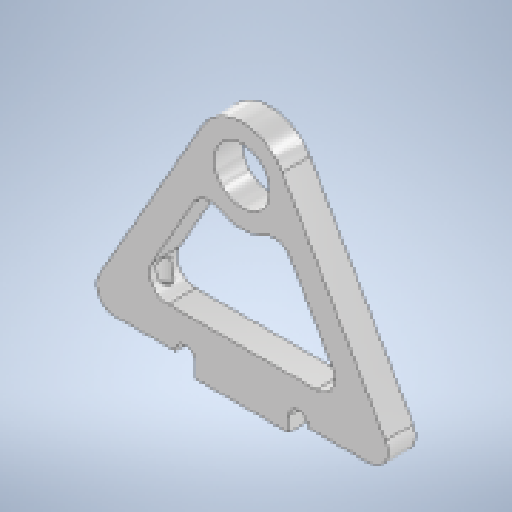
# Autodesk Inventor part: kosipiti
Saved by Autodesk Inventor 2025.1 (Build 291241000, 241)
## iProperties
Created: 2024-09-01
Part Number: kosipiti
Material: アルミニウム 2014-T4
Document SubType Name: Modeling
Designer: right
Density: 2.8 g/cm^3
Appearance: サテン
Mass: 2.87521 g
Surface Area: 14.5004 cm^2
Volume: 1.02686 cm^3
Author: right
Autodesk Inventor part; units mm, degrees
ref_plane "YZ Plane" through (0, 0, 0) normal (1, 0, 0) x (0, 1, 0)
ref_plane "XZ Plane" through (0, 0, 0) normal (0, 1, 0) x (-1, 0, 0)
ref_plane "XY Plane" through (0, 0, 0) normal (0, 0, 1) x (1, 0, 0)
sketch "スケッチ1" plane through (0, 0, 0) normal (0, 0, 1) x (1, 0, 0)
  circle A0 centre (0, 0) radius 3
  circle A1 centre (0, 0) radius 5
  line L0 (-5, -20) -> (5, -20)
  line L1 (5, -20) -> (5, -21.5)
  line L2 (5, -21.5) -> (-5, -21.5)
  line L3 (-5, -21.5) -> (-5, -20)
  circle A2 centre (-6.1, -20) radius 1.1
  line L4 (0, 0) -> (0, -20) construction
  circle A3 centre (6.1, -20) radius 1.1
  line L5 (-7.2, -20) -> (-17.2, -20)
  line L6 (-17.2, -20) -> (-4.3402, 2.4825)
  line L7 (7.2, -20) -> (17.2, -20)
  line L8 (17.2, -20) -> (4.3402, 2.4825)
  point P0 (0, -21.5)
  point P1 (4.3402, 2.4825)
  dimension "d1" = 10
  dimension "d0" = 6
  dimension "d2" = 10
  dimension "d3" = 1.5
  dimension "d4" = 2.2
  dimension "d5" = 20
  dimension "d6" = 10
  constraints: 18 end point, 4 symmetric about line, 3 centre point, 2 coincident, 2 horizontal, 2 horizontal alignment, 2 midpoint, 2 parallel, 2 point on circle, 1 perpendicular, 1 vertical alignment, 5 other
  measures "d0" diameter of A0
  measures "d2" distance of L1.end L2.end
  measures "d3" distance of L0.end L1.end
  measures "d4" diameter of A2
  measures "d5" distance from line of L0 L4.start
  measures "d6" distance of L5.start L5.end
extrude "押し出し1" add sketch "スケッチ1" along normal blind 3 contours A1 | A1 L8 L7 A3 L0 A2 L5 L6 | L1 L2 L3 L0
fillet "フィレット1" radius 2 2 edges at (-17.2, -20, 1.5) (17.2, -20, 1.5)
sketch "スケッチ3" plane through (0, 0, 0) normal (0, 0, -1) x (-1, 0, 0)
  arc A0 (-15.488, -17.007) -> (-13.752, -20) centre (-13.752, -18) ccw projected
  line L0 (-7.2, -20) -> (-13.752, -20) projected
  arc A1 (-5, -20) -> (-7.2, -20) centre (-6.1, -20) ccw projected
  line L1 (-5, -21.5) -> (-5, -20) projected
  line L2 (5, -21.5) -> (-5, -21.5) projected
  line L3 (5, -20) -> (5, -21.5) projected
  arc A2 (7.2, -20) -> (5, -20) centre (6.1, -20) ccw projected
  line L4 (13.752, -20) -> (7.2, -20) projected
  arc A3 (13.752, -20) -> (15.488, -17.007) centre (13.752, -18) ccw projected
  line L5 (4.3402, 2.4825) -> (15.488, -17.007) projected
  arc A4 (4.3402, 2.4825) -> (-4.3402, 2.4825) centre (0, 0) ccw projected
  line L6 (-15.488, -17.007) -> (-4.3402, 2.4825) projected
  circle A5 centre (0, 0) radius 3 projected
  line L7 (-11.4559, -16) -> (11.4559, -16)
  line L8 (11.4559, -16) -> (4.0113, -2.9848)
  line L9 (-11.4559, -16) -> (-4.0113, -2.9848)
  line L10 (-15.488, -17.007) -> (-4.3402, 2.4825) projected
  circle A6 centre (0, 0) radius 5
  line L11 (5, -21.5) -> (-5, -21.5) projected
  arc A7 (4.3402, 2.4825) -> (-4.3402, 2.4825) centre (0, 0) ccw projected
  point P0 (0, -21.5)
  point P1 (0, -16)
  point P2 (0, -21.5)
  dimension "d19" = 4
  dimension "d20" = 3
  constraints: 6 end point, 3 midpoint, 3 parallel, 2 point on circle, 2 vertical alignment, 1 centre point, 1 coincident, 1 concentric, 1 horizontal
  measures "d19" distance from line of A2.centre L7
  measures "d20" distance between parallel lines of L6 L9
extrude "押し出し2" cut sketch "スケッチ3" against normal through all contours A6 L8 L7 L9
fillet "フィレット2" radius 2 4 edges at (-4.0113, -2.9848, 1.5) (4.0113, -2.9848, 1.5) (-11.4559, -16, 1.5) (11.4559, -16, 1.5)
sketch "スケッチ2" plane through (-17.2, -20, 0) normal (0, -1, 0) x (1, 0, 0)
  line L0 (12.2, 0) -> (12.2, 3) projected
  line L1 (22.2, 0) -> (22.2, 3) projected
  point P0 (17.2, 0)
  point P1 (7.2, 1.5)
  point P2 (27.2, 1.5)
  point P3 (12.2, 1.5)
  point P4 (22.2, 1.5)
  point P5 (12.2, 1.5)
  point P6 (22.2, 1.5)
  dimension "d9" = 5
  dimension "d10" = 5
  constraints: 4 midpoint, 2 horizontal alignment
  measures "d9" distance of point (7.2, 1.5) point (12.2, 1.5)
  measures "d10" distance of point (27.2, 1.5) point (22.2, 1.5)
hole "穴1" at (-10, -20, 1.5) at (10, -20, 1.5) direction (0, 1, 0) diameter 1.567 depth 6.3 tip angle 118 thread size "M2x0.4" class "6H" standard "ISO Metric profile"
sketch "スケッチ4" plane through (0, 0, 0) normal (0, 0, -1) x (-1, 0, 0)
  line L0 (5.405, -15.9) -> (-14.4109, -15.9) construction
  arc A0 (-15.5215, -12.2367) -> (-14.4109, -15.9) centre (-14.4109, -13.9) ccw construction
  line L1 (-15.5215, -12.2367) -> (-4.1487, -4.643) construction
  arc A1 (-2.1701, -4.5045) -> (-4.1487, -4.643) centre (-3.0381, -6.3063) ccw construction
  arc A2 (-2.1701, -4.5045) -> (2.4825, -4.3402) centre (0, 0) ccw construction
  arc A3 (5.2116, -5.0832) -> (2.4825, -4.3402) centre (3.4756, -6.0762) ccw construction
  line L2 (5.2116, -5.0832) -> (7.3308, -8.7882) construction
  arc A4 (7.377, -10.6888) -> (7.3308, -8.7882) centre (5.5948, -9.7812) ccw projected
  arc A5 (7.377, -10.6888) -> (7.2631, -13.1601) centre (10.0503, -12.0503) ccw projected
  arc A6 (5.405, -15.9) -> (7.2631, -13.1601) centre (5.405, -13.9) ccw projected
  line L3 (4.3402, 2.4825) -> (9.529, -6.589) construction
  arc A7 (4.3402, 2.4825) -> (0, 5) centre (0, 0) ccw construction
  line L4 (-8, 5) -> (0, 5) construction
  arc A8 (-8, 5) -> (-10.7765, 4.1583) centre (-8, 0) ccw construction
  line L5 (-33.2416, -10.8417) -> (-10.7765, 4.1583) construction
  arc A9 (-33.2416, -10.8417) -> (-30.4651, -20) centre (-30.4651, -15) ccw construction
  line L6 (-7.2, -20) -> (-30.4651, -20) construction
  arc A10 (-5, -20) -> (-7.2, -20) centre (-6.1, -20) ccw construction
  line L7 (-5, -21.5) -> (-5, -20) construction
  line L8 (5, -21.5) -> (-5, -21.5) construction
  line L9 (5, -20) -> (5, -21.5) construction
  arc A11 (7.2, -20) -> (5, -20) centre (6.1, -20) ccw construction
  line L10 (15, -20) -> (7.2, -20) projected
  arc A12 (15, -20) -> (17.1213, -19.1213) centre (15, -17) ccw projected
  line L11 (17.1213, -19.1213) -> (22.0711, -14.1716) projected
  arc A13 (22.0711, -14.1716) -> (22.0711, -9.9289) centre (19.9497, -12.0503) ccw projected
  arc A14 (22.0711, -9.9289) -> (11.8876, -7.4967) centre (15, -17) ccw projected
  arc A15 (9.529, -6.589) -> (11.8876, -7.4967) centre (11.2651, -5.596) ccw projected
  arc A16 (9.2724, -11.2724) -> (10.8281, -12.8281) centre (10.0503, -12.0503) ccw projected
  arc A17 (20.7276, -11.2724) -> (9.2724, -11.2724) centre (15, -17) ccw projected
  arc A18 (19.1719, -12.8281) -> (20.7276, -11.2724) centre (19.9497, -12.0503) ccw projected
  arc A19 (19.1719, -12.8281) -> (10.8281, -12.8281) centre (15, -17) ccw projected
  line L12 (-9.6659, 2.495) -> (-32.131, -12.505) construction
  arc A20 (-6.3341, -2.495) -> (-9.6659, 2.495) centre (-8, 0) ccw construction
  line L13 (-28.7992, -17.495) -> (-6.3341, -2.495) construction
  arc A21 (-32.131, -12.505) -> (-28.7992, -17.495) centre (-30.4651, -15) ccw construction
  circle A22 centre (0, 0) radius 3 construction
  circle A23 centre (15, -17) radius 1.1 projected
  line L14 (5.405, -15.9) -> (5.405, -16)
  line L15 (8.0079, -16) -> (-8.0079, -16) projected
  arc A24 (-2.4825, -4.3402) -> (2.4825, -4.3402) centre (0, 0) ccw projected
  arc A25 (5.2116, -5.0832) -> (2.4825, -4.3402) centre (3.4756, -6.0762) ccw projected
  line L16 (5.2116, -5.0832) -> (9.744, -13.007) projected
  arc A26 (8.0079, -16) -> (9.744, -13.007) centre (8.0079, -14) ccw projected
  line L17 (8.0079, -16) -> (-8.0079, -16) projected
  arc A27 (-9.744, -13.007) -> (-8.0079, -16) centre (-8.0079, -14) ccw projected
  line L18 (-9.744, -13.007) -> (-5.2116, -5.0832) projected
  arc A28 (-2.4825, -4.3402) -> (-5.2116, -5.0832) centre (-3.4756, -6.0762) ccw projected
  arc A29 (-15.488, -17.007) -> (-13.752, -20) centre (-13.752, -18) ccw projected
  line L19 (-7.2, -20) -> (-13.752, -20) projected
  arc A30 (-5, -20) -> (-7.2, -20) centre (-6.1, -20) ccw projected
  line L20 (-5, -21.5) -> (-5, -20) projected
  line L21 (5, -21.5) -> (-5, -21.5) projected
  line L22 (5, -20) -> (5, -21.5) projected
  arc A31 (7.2, -20) -> (5, -20) centre (6.1, -20) ccw projected
  line L23 (13.752, -20) -> (7.2, -20) projected
  arc A32 (13.752, -20) -> (15.488, -17.007) centre (13.752, -18) ccw projected
  line L24 (4.3402, 2.4825) -> (15.488, -17.007) projected
  arc A33 (4.3402, 2.4825) -> (-4.3402, 2.4825) centre (0, 0) ccw projected
  line L25 (-15.488, -17.007) -> (-4.3402, 2.4825) projected
  circle A34 centre (0, 0) radius 3 projected
  point P0 (9.529, -6.589)
  point P1 (11.3484, -9.7698)
  point P2 (12.4427, -11.683)
  point P3 (14.86, -15.909)
  point P4 (15.743, -17.8111)
  point P5 (9.8052, -13.1226)
  point P6 (9.0034, -11.7124)
  point P7 (7.3308, -8.7882)
  constraints: 2 end point, 1 point on line, 1 vertical
sketch "スケッチ5" plane through (0, 0, 0) normal (0, 0, -1) x (-1, 0, 0)
  circle A0 centre (15, -17) radius 2 projected
  arc A1 (20.7276, -11.2724) -> (9.2724, -11.2724) centre (15, -17) ccw projected
  arc A2 (9.2724, -11.2724) -> (10.8281, -12.8281) centre (10.0503, -12.0503) ccw projected
  arc A3 (19.1719, -12.8281) -> (10.8281, -12.8281) centre (15, -17) ccw projected
  arc A4 (19.1719, -12.8281) -> (20.7276, -11.2724) centre (19.9497, -12.0503) ccw projected
  arc A5 (18.5355, -13.4645) -> (11.4645, -13.4645) centre (15, -17) ccw projected
  arc A6 (8.636, -10.636) -> (11.4645, -13.4645) centre (10.0503, -12.0503) ccw projected
  arc A7 (21.364, -10.636) -> (8.636, -10.636) centre (15, -17) ccw projected
  arc A8 (18.5355, -13.4645) -> (21.364, -10.636) centre (19.9497, -12.0503) ccw projected
  point P0 (0, 0)
equation "\"d10\" = d9"
